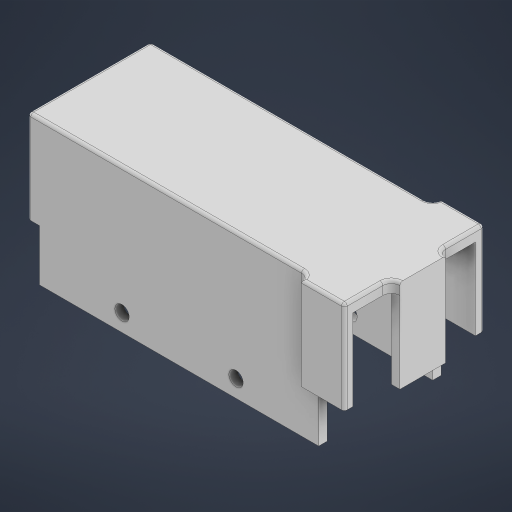
# Autodesk Inventor part: carcasa_baterias
Saved by Autodesk Inventor 2023.1 (Build 271208000, 208)
## iProperties
Created: 2022-11-10
Part Number: carcasa_baterias
Material: Generic
Document SubType Name: Modeling
Designer: amtat
Density: 1 g/cm^3
Appearance: Default
Author: amtat
Autodesk Inventor part; units mm, degrees
ref_plane "YZ Plane" through (0, 0, 0) normal (1, 0, 0) x (0, 1, 0)
ref_plane "XZ Plane" through (0, 0, 0) normal (0, 1, 0) x (-1, 0, 0)
ref_plane "XY Plane" through (0, 0, 0) normal (0, 0, 1) x (1, 0, 0)
sketch "Sketch1" plane through (0, 0, 0) normal (1, 0, 0) x (0, 1, 0)
  line L0 (0, 0) -> (0, -3)
  line L1 (0, -3) -> (4.1852, -3)
  line L2 (0, 0) -> (4.1852, 0)
  line L3 (0, -3) -> (0, -4)
  line L4 (0, -4) -> (0, -39)
  line L5 (0, -39) -> (0, -40)
  line L6 (0, -40) -> (0, -43)
  line L7 (0, -40) -> (28.5, -40)
  line L8 (28.5, -40) -> (28.5, -43)
  line L9 (28.5, -43) -> (0, -43)
  line L10 (0, -3) -> (28.5, -3)
  line L11 (28.5, -3) -> (28.5, 0)
  line L12 (28.5, 0) -> (0, 0)
  dimension "d0" = 3
  dimension "d1" = 1
  dimension "d2" = 35
  dimension "d3" = 1
  dimension "d4" = 3
  dimension "d5" = 28.5
  dimension "d6" = 28.5
  constraints: 26 end point, 4 perpendicular, 3 horizontal, 3 point on line, 2 vertical, 1 collinear
  measures "d0" distance of L0.start L0.end
  measures "d1" distance of L0.end L3.end
  measures "d2" distance of L3.end L4.end
  measures "d3" distance of L4.end L5.end
  measures "d4" distance of L5.end L6.end
  measures "d5" distance of L5.end L7.end
  measures "d6" distance of L0.end L10.end
extrude "Extrusion1" add sketch "Sketch1" along normal blind 98
sketch "Sketch2" plane through (0, 0, -43) normal (0, 0, -1) x (-1, 0, 0)
  line L0 (0, 0) -> (0, 28.5) projected
  line L1 (0, 28.5) -> (0, 0) projected
  line L2 (0, 28.5) -> (4, 28.5)
  line L3 (4, 28.5) -> (4, 0)
  line L4 (4, 0) -> (0, 0)
  dimension "d9" = 4
  constraints: 6 end point, 2 perpendicular, 1 horizontal
  measures "d9" distance of L0.end L2.end
extrude "Extrusion2" add sketch "Sketch2" against normal blind 43
sketch "Sketch3" plane through (98, 0, -43) normal (0, 0, -1) x (-1, 0, 0)
  line L0 (102, 28.5) -> (0, 28.5) projected
  line L1 (0, 0) -> (0, 28.5) projected
  line L2 (0, 0) -> (102, 0) projected
  line L3 (102, 0) -> (102, 28.5) projected
  line L4 (102, 28.5) -> (0, 28.5) projected
  line L5 (0, 28.5) -> (3, 28.5)
  line L6 (3, 28.5) -> (3, 0)
  line L7 (98, 0) -> (0, 0) projected
  point P0 (3, 28.5)
  dimension "d12" = 3
  constraints: 4 end point, 2 point on line, 1 perpendicular
  measures "d12" distance of L0.end L5.end
extrude "Extrusion3" add sketch "Sketch3" along normal blind 3 contours L6 L2 L1 L0
sketch "Sketch4" plane through (98, 0, 0) normal (0, 0, 1) x (1, 0, 0)
  line L0 (0, 0) -> (-3, 0) projected
  line L1 (-3, 0) -> (-3, 28.5) projected
  line L2 (-3, 28.5) -> (0, 28.5) projected
  line L3 (0, 28.5) -> (0, 0) projected
  point P0 (-98, 0)
extrude "Extrusion4" add sketch "Sketch4" along normal blind 3
sketch "Sketch5" plane through (98, 0, 0) normal (1, 0, 0) x (0, 0, -1)
  line L0 (3, 0) -> (3, 28.5) projected
  line L1 (3, 28.5) -> (-3, 28.5) projected
  line L2 (-3, 0) -> (-3, 28.5) projected
  line L3 (3, 0) -> (-3, 0) projected
  line L4 (40, 28.5) -> (46, 28.5) projected
  line L5 (40, 28.5) -> (40, 0) projected
  line L6 (40, 0) -> (46, 0) projected
  line L7 (46, 28.5) -> (46, 0) projected
  line L8 (3, 28.5) -> (-3, 28.5) projected
  line L9 (-3, 28.5) -> (0, 28.5)
  line L10 (0, 28.5) -> (0, 0)
  line L11 (43, 0) -> (43, 28.5) projected
  line L12 (43, 28.5) -> (43, 0)
  line L13 (43, 0) -> (46, 0)
  constraints: 8 end point, 1 collinear, 1 midpoint, 1 perpendicular, 1 vertical
extrude "Extrusion5" add sketch "Sketch5" along normal blind 12 contours L3 L2 L1 L10 | L4 L7 L6 L11
sketch "Sketch6" plane through (0, 28.5, -40) normal (0, 1, 0) x (1, 0, 0)
  line L0 (0, 0) -> (98, 0) projected
  line L1 (98, 0) -> (98, 3) projected
  line L2 (98, 3) -> (110, 3) projected
  line L3 (110, 6) -> (110, 3) projected
  line L4 (95, 6) -> (110, 6) projected
  line L5 (95, 3) -> (95, 6) projected
  line L6 (-4, 3) -> (95, 3) projected
  line L7 (-4, 3) -> (-4, -40) projected
  line L8 (-4, -40) -> (95, -40) projected
  line L9 (95, -40) -> (95, -43) projected
  line L10 (95, -43) -> (110, -43) projected
  line L11 (110, -40) -> (110, -43) projected
  line L12 (98, -40) -> (110, -40) projected
  line L13 (98, -37) -> (98, -40) projected
  line L14 (0, -37) -> (98, -37) projected
  line L15 (0, 0) -> (0, -37) projected
  line L16 (98, -40) -> (110, -40) projected
  line L17 (110, 3) -> (110, 6) projected
  line L18 (110, -40) -> (110, 3)
  point P0 (0, -40)
  constraints: 2 end point, 1 vertical
extrude "Extrusion6" add sketch "Sketch6" along normal blind 4
sketch "Sketch7" plane through (0, 28.5, -40) normal (0, -1, 0) x (1, 0, 0)
  line L0 (98, 40) -> (110, 40) projected
  line L1 (98, 37) -> (98, 40) projected
  line L2 (0, 37) -> (98, 37) projected
  line L3 (0, 0) -> (0, 37) projected
  line L4 (0, 0) -> (98, 0) projected
  line L5 (98, 0) -> (98, -3) projected
  line L6 (98, -3) -> (110, -3) projected
  line L7 (110, 40) -> (110, -3) projected
  line L8 (110, 40) -> (110, -3) projected
  line L9 (110, 40) -> (110, 18.5)
  line L10 (110, 18.5) -> (110, 10.5)
  line L11 (110, 18.5) -> (110, 26.5)
  line L12 (110, 26.5) -> (113, 26.5)
  line L13 (113, 26.5) -> (113, 18.5)
  line L14 (113, 18.5) -> (113, 10.5)
  line L15 (113, 10.5) -> (110, 10.5)
  point P0 (0, 40)
  point P1 (110, 10.5)
  dimension "d21" = 21.5
  dimension "d22" = 8
  dimension "d23" = 8
  dimension "d24" = 3
  constraints: 14 end point, 3 perpendicular, 2 point on line, 1 midpoint, 1 vertical
  measures "d21" distance of L0.end L9.end
  measures "d22" distance of L9.end L10.end
  measures "d23" distance of L9.end L11.end
  measures "d24" distance of L11.end L12.end
extrude "Extrusion7" add sketch "Sketch7" along normal blind 28.5 contours L12 L13 L14 L15 L7
sketch "Sketch8" plane through (110, 0, 0) normal (1, 0, 0) x (0, 0, -1)
  line L0 (-3, 0) -> (0, 0) projected
  line L1 (0, 0) -> (0, 28.5) projected
  line L2 (0, 28.5) -> (13.5, 28.5) projected
  line L3 (13.5, 28.5) -> (29.5, 28.5) projected
  line L4 (29.5, 28.5) -> (43, 28.5) projected
  line L5 (43, 28.5) -> (43, 0) projected
  line L6 (43, 0) -> (46, 0) projected
  line L7 (46, 0) -> (46, 32.5) projected
  line L8 (-3, 32.5) -> (46, 32.5) projected
  line L9 (-3, 0) -> (-3, 32.5) projected
  line L10 (29.5, 28.5) -> (13.5, 28.5) projected
  line L11 (13.5, 28.5) -> (29.5, 28.5) projected
  line L12 (13.5, 28.5) -> (13.5, 32.5)
  line L13 (-3, 32.5) -> (46, 32.5) projected
  line L14 (29.5, 28.5) -> (43, 28.5) projected
  line L15 (29.5, 28.5) -> (29.5, 32.5)
  constraints: 4 end point, 2 point on line, 1 parallel, 1 perpendicular
extrude "Extrusion8" add sketch "Sketch8" along normal blind 3 contours L8 L15 L3 L12
sketch "Sketch9" plane through (0, 0, -40) normal (0, -1, 0) x (1, 0, 0)
  line L0 (98, 0) -> (98, -3) projected
  line L1 (0, 0) -> (98, 0) projected
  line L2 (0, 0) -> (0, 37) projected
  line L3 (0, 37) -> (98, 37) projected
  line L4 (98, 37) -> (98, 40) projected
  line L5 (98, 40) -> (110, 40) projected
  line L6 (110, 43) -> (110, 40) projected
  line L7 (95, 43) -> (110, 43) projected
  line L8 (95, 40) -> (95, 43) projected
  line L9 (-4, 40) -> (95, 40) projected
  line L10 (-4, -3) -> (-4, 40) projected
  line L11 (95, -3) -> (-4, -3) projected
  line L12 (95, -3) -> (95, -6) projected
  line L13 (95, -6) -> (110, -6) projected
  line L14 (110, -3) -> (110, -6) projected
  line L15 (98, -3) -> (110, -3) projected
  line L16 (95, -3) -> (-4, -3) projected
  line L17 (98, -3) -> (110, -3) projected
  line L18 (95, -3) -> (98, -3)
  line L19 (0, 0) -> (98, 0) projected
  line L20 (0, 0) -> (0, -3)
  line L21 (0, 37) -> (0, 40)
  line L22 (95, 40) -> (95, 43) projected
  line L23 (98, 37) -> (98, 40) projected
  line L24 (95, 40) -> (98, 40)
  constraints: 8 end point, 2 horizontal, 1 perpendicular, 1 point on line, 1 vertical
extrude "Extrusion9" add sketch "Sketch9" along normal blind 18 contours L0 L18 L11 L20 L1 | L21 L9 L24 L4 L3
sketch "Sketch10" plane through (-4, 0, -43) normal (0, 0, -1) x (-1, 0, 0)
  line L0 (-99, 32.5) -> (-99, 0) projected
  line L1 (-102, 0) -> (-99, 0) projected
  line L2 (-102, 0) -> (-102, -18) projected
  line L3 (-4, -18) -> (-102, -18) projected
  line L4 (-4, 0) -> (-4, -18) projected
  line L5 (-4, 0) -> (0, 0) projected
  line L6 (0, 0) -> (0, 32.5) projected
  line L7 (-99, 32.5) -> (0, 32.5) projected
  line L8 (-4, 0) -> (-4, -18) projected
  line L9 (-4, -18) -> (-53, -18)
  line L10 (-53, -18) -> (-73, -18)
  line L11 (-4, -18) -> (-102, -18) projected
  line L12 (-73, -18) -> (-73, -12)
  circle A0 centre (-73, -12) radius 2.5
  line L13 (-53, -18) -> (-53, -7.624)
  circle A1 centre (-33, -12) radius 2.5
  dimension "d31" = 49
  dimension "d32" = 20
  dimension "d33" = 6
  dimension "d34" = 5
  constraints: 8 end point, 2 centre point, 1 coincident, 1 midpoint, 1 perpendicular, 1 point on line, 1 symmetric about line, 1 vertical, 1 other
  measures "d31" distance of L3.start L9.end
  measures "d32" distance of L9.end L10.end
  measures "d33" distance of L10.end L12.end
  measures "d34" diameter of A0
extrude "Extrusion10" cut sketch "Sketch10" against normal through all contours A0 | A1
fillet "Fillet1" radius 3 4 edges at (95, 16.25, -43) (110, 30.5, -29.5) (110, 30.5, -13.5) (95, 16.25, 0)
fillet "Fillet2" radius 1 4 edges at (98, 14.25, 0) (0, 14.25, -3) (98, 14.25, -43) (0, 14.25, -40)
fillet "Fillet3" radius 1 14 edges at (-4, 16.25, -43) (95, 32.5, -45.9999) (44.0001, 32.5, -43) (-4, 32.5, -21.5) (95, 32.5, 2.9999) (44.0001, 32.5, 0) (-4, 16.25, 0) (102.5, 32.5, -46) (102.5, 32.5, 3) (110.8787, 32.5, -12.6213) (110, 32.5, -39.2499) (110.8787, 32.5, -30.3787) (110, 16.25, -46) (110, 16.25, 3)
fillet "Fillet4" radius 1 5 edges at (0.2929, 28.5, -3.2929) (0, 28.5, -21.5) (0.2929, 28.5, -39.7071) (49.5, 28.5, -40) (49.5, 28.5, -3)
body "Solid1"
